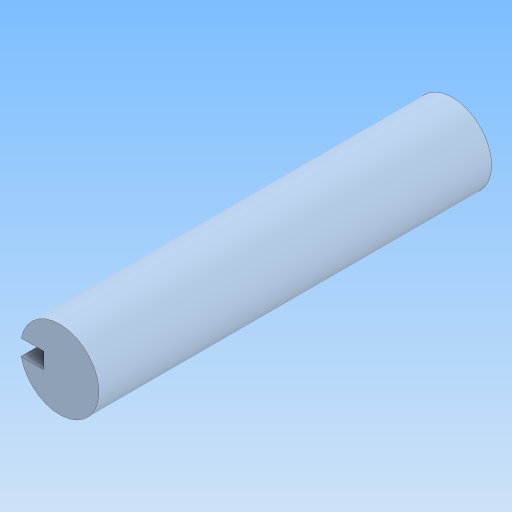
# Autodesk Inventor part: Welle_000
Saved by Autodesk Inventor 2024.4 (Build 284460000, 460)
## iProperties
Created: 2026-01-21
Part Number: Welle_000
Material: Generisch
Document SubType Name: Modeling
Designer: windows-desktop
Density: 1 g/cm^3
Appearance: Vorgabe
Mass: 101.073 g
Surface Area: 166.155 cm^2
Volume: 101.073 cm^3
Masse[kg]: 0,101 kg
Author: windows-desktop
Autodesk Inventor part; units mm, degrees
ref_plane "YZ Plane" through (0, 0, 0) normal (1, 0, 0) x (0, 1, 0)
ref_plane "XZ Plane" through (0, 0, 0) normal (0, 1, 0) x (-1, 0, 0)
ref_plane "XY Plane" through (0, 0, 0) normal (0, 0, 1) x (1, 0, 0)
sketch "Skizze1" plane through (0, 0, 0) normal (0, 1, 0) x (-1, 0, 0)
  circle A0 centre (0, 0) radius 15
  dimension "d0" = 30
  constraints: 1 centre point, 1 coincident
  measures "d0" diameter of A0
extrude "Extrusion1" add sketch "Skizze1" along normal blind 150
sketch "Skizze2" plane through (0, 150, 0) normal (0, 1, 0) x (1, 0, 0)
  line L0 (-16, -5) -> (-6, -5)
  line L1 (-6, -5) -> (-6, 5)
  line L2 (-6, 5) -> (-16, 5)
  line L3 (-16, 5) -> (-16, -5)
  line L4 (-22.2, 0) -> (21.2, 0) construction
  line L5 (0, 21) -> (0, -21) construction
  dimension "d3" = 6
  dimension "d4" = 10
  dimension "d5" = 10
  constraints: 8 end point, 2 parallel, 1 horizontal, 1 perpendicular, 1 other
  measures "d3" distance between parallel lines of L5 L1
  measures "d4" distance of L1.end L2.end
  measures "d5" distance of L2.end L0.start
extrude "Extrusion2" cut sketch "Skizze2" against normal blind 44.6
sketch "Skizze3" plane through (0, 0, 0) normal (0, -1, 0) x (1, 0, 0)
  line L0 (-18, -3) -> (-6, -3)
  line L1 (-6, -3) -> (-6, 3)
  line L2 (-6, 3) -> (-18, 3)
  line L3 (-18, 3) -> (-18, -3)
  line L4 (-24.6, 0) -> (21.6, 0) construction
  line L5 (0, -21) -> (0, 21) construction
  dimension "d8" = 6
  dimension "d9" = 12
  dimension "d10" = 6
  constraints: 8 end point, 2 parallel, 1 horizontal, 1 perpendicular, 1 other
  measures "d8" distance between parallel lines of L5 L1
  measures "d9" distance of L1.end L2.end
  measures "d10" distance of L2.end L0.start
extrude "Extrusion3" cut sketch "Skizze3" against normal blind 20
